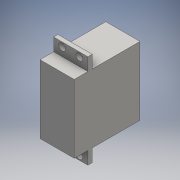
# Autodesk Inventor part: servo
Saved by Autodesk Inventor 2016 (Build 200138000, 138)
## iProperties
Created: 2016-04-14
Part Number: servo
Material: Generic
Document SubType Name: Modeling
Designer: hesaon
Density: 1 g/cm^3
Appearance: Default
Author: hesaon
Autodesk Inventor part; units mm, degrees
ref_plane "YZ Plane" through (0, 0, 0) normal (1, 0, 0) x (0, 1, 0)
ref_plane "XZ Plane" through (0, 0, 0) normal (0, 1, 0) x (-1, 0, 0)
ref_plane "XY Plane" through (0, 0, 0) normal (0, 0, 1) x (1, 0, 0)
sketch "Sketch4" plane through (0, 0, 0) normal (0, 1, 0) x (-1, 0, 0)
  line L0 (0, 0) -> (20, 0)
  line L1 (20, 0) -> (20, -20)
  line L2 (20, -20) -> (0, -20)
  line L3 (0, -20) -> (0, 0)
  dimension "d16" = 20
  dimension "d17" = 20
  constraints: 8 end point, 2 parallel, 1 horizontal, 1 perpendicular
  measures "d16" distance of L1.end L2.end
  measures "d17" distance of L0.end L1.end
extrude "Extrusion4" add sketch "Sketch4" along normal blind 38.5
sketch "Sketch5" plane through (-20, 0, 0) normal (0, 0, 1) x (1, 0, 0)
  line L0 (0, 0) -> (0, 38.5) projected
  line L1 (20, 0) -> (20, 38.5) projected
  line L2 (0, 10.5) -> (20, 10.5)
  line L3 (20, 10.5) -> (20, 8)
  line L4 (20, 8) -> (0, 8)
  line L5 (0, 8) -> (0, 10.5)
  dimension "d20" = 2.5
  dimension "d21" = 8
  constraints: 8 end point, 2 parallel, 2 point on line, 1 horizontal, 1 perpendicular
  measures "d20" distance of L2.end L3.end
  measures "d21" distance of L1.start L3.end
extrude "Extrusion5" add sketch "Sketch5" along normal blind 7.5
sketch "Sketch6" plane through (-20, 10.5, 0) normal (0, 1, 0) x (1, 0, 0)
  circle A0 centre (5, -5) radius 2
  circle A1 centre (15, -5) radius 2
  line L0 (0, 0) -> (20, 0) projected
  line L1 (0, 0) -> (0, -7.5) projected
  line L2 (20, 0) -> (20, -7.5) projected
  dimension "d24" = 4
  dimension "d25" = 4
  dimension "d26" = 5
  dimension "d27" = 5
  dimension "d28" = 5
  dimension "d29" = 5
  constraints: 2 centre point
  measures "d24" diameter of A0
  measures "d25" diameter of A1
  measures "d26" distance from line of L0 A0.centre
  measures "d27" distance from line of L0 A1.centre
  measures "d28" distance from line of L1 A0.centre
  measures "d29" distance from line of L2 A1.centre
extrude "Extrusion6" cut sketch "Sketch6" against normal through all
mirror "Mirror1" about plane through (0, 0, -20) normal (0, 0, -1)
body "Solid2"
